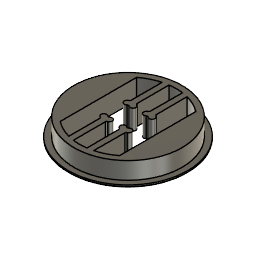
shifter bracket_v1 (Autodesk Fusion 360 design; units mm, degrees)
Autodesk Fusion 360 part; units mm, degrees
note: some values were not read from the file. Set by a fixed rule: which sketch regions a step uses.
sketch "Sketch1" plane through (0, 0, 0) normal (0, 0, 1) x (1, 0, 0)
  circle A0 centre (0, 0) radius 21
  dimension "d1" = 42
  constraint coincident A0.centre origin
  measures "d1" diameter of A0
extrude "Extrude1" add sketch "Sketch1" along normal blind 1
sketch "Sketch2" plane through (0, 0, 1) normal (0, 0, 1) x (-1, 0, 0)
  circle A0 centre (0, 0) radius 21
  circle A1 centre (0, 0) radius 19
  dimension "d4" = 38
  constraint coincident A0.centre A1.centre
  measures "d4" diameter of A1
extrude "Extrude2" add sketch "Sketch2" along normal blind 6 contours A1
sketch "Sketch3" plane through (0, 0, 7) normal (0, 0, 1) x (-1, 0, 0)
  circle A0 centre (0, 0) radius 19
  circle A1 centre (0, 0) radius 2 construction
  line L0 (4.4074, 16.8232) -> (4.4074, 5.4989)
  line L1 (2.372, 5.5528) -> (2.372, 17.2616)
  line L2 (0, 0) -> (0, 17.8293) construction
  line L3 (-4.3475, 16.841) -> (-4.4034, 5.4975)
  line L4 (-2.3033, 5.524) -> (-2.372, 17.2616)
  arc A2 (-3.0182, 3.3969) -> (-1.9879, 5.0695) centre (-2.3432, 4.1347) ccw
  arc A3 (-4.736, 5.035) -> (-3.7057, 3.3816) centre (-4.413, 4.0885) ccw
  arc A4 (3.7057, 3.3816) -> (4.7389, 5.034) centre (4.413, 4.0885) ccw
  arc A5 (2.0329, 5.0854) -> (3.0182, 3.3969) centre (2.3432, 4.1347) ccw
  line L5 (8.974, 0) -> (-11.026, 0) construction
  line L6 (-10.4146, 13.4129) -> (-10.4146, -13.4129)
  circle A6 centre (0, 0) radius 2 construction
  line L7 (10.4146, 13.4129) -> (10.4146, -13.4129)
  arc A7 (-3.0182, 3.3969) -> (-3.7057, 3.3816) centre (-3.354, 3.03) ccw
  arc A8 (-2.3033, 5.524) -> (-1.9879, 5.0695) centre (-1.8141, 5.5268) ccw
  arc A9 (-4.736, 5.035) -> (-4.4034, 5.4975) centre (-4.8947, 5.4999) ccw
  arc A10 (2.0329, 5.0854) -> (2.372, 5.5528) centre (1.8803, 5.5528) ccw
  arc A11 (3.7057, 3.3816) -> (3.0182, 3.3969) centre (3.354, 3.03) ccw
  arc A12 (4.4074, 5.4989) -> (4.7389, 5.034) centre (4.8991, 5.4989) ccw
  arc A13 (-4.4034, -5.4975) -> (-4.736, -5.035) centre (-4.8947, -5.4999) ccw
  arc A14 (-1.9879, -5.0695) -> (-3.0182, -3.3969) centre (-2.3432, -4.1347) ccw
  arc A15 (-1.9879, -5.0695) -> (-2.3033, -5.524) centre (-1.8141, -5.5268) ccw
  arc A16 (3.0182, -3.3969) -> (2.0329, -5.0854) centre (2.3432, -4.1347) ccw
  arc A17 (3.0182, -3.3969) -> (3.7057, -3.3816) centre (3.354, -3.03) ccw
  arc A18 (4.7389, -5.034) -> (3.7057, -3.3816) centre (4.413, -4.0885) ccw
  arc A19 (-3.7057, -3.3816) -> (-4.736, -5.035) centre (-4.413, -4.0885) ccw
  arc A20 (2.372, -5.5528) -> (2.0329, -5.0854) centre (1.8803, -5.5528) ccw
  arc A21 (-3.7057, -3.3816) -> (-3.0182, -3.3969) centre (-3.354, -3.03) ccw
  arc A22 (4.7389, -5.034) -> (4.4074, -5.4989) centre (4.8991, -5.4989) ccw
  line L8 (4.4074, -16.8232) -> (4.4074, -5.4989)
  line L9 (2.372, -5.5528) -> (2.372, -17.2616)
  line L10 (-2.3033, -5.524) -> (-2.372, -17.2616)
  line L11 (-4.3475, -16.841) -> (-4.4034, -5.4975)
  circle A23 centre (0, 0) radius 16.9815
  point P0 (0, 10.0735)
  point P1 (0, -10.0735)
  dimension "d7" = 4
  dimension "d9" = 2
  dimension "d14" = 2
  constraint coincident A0.centre A1.centre
  constraint vertical L0
  constraint vertical L1
  constraint vertical L2
  constraint coincident L2 P0
  constraint symmetric L1.end L2 L4.end
  constraint symmetric L2 A2 A5
  constraint symmetric L2 A3 A4
  constraint horizontal L5
  constraint vertical L6
  constraint symmetric A1 L2 A6
  constraint symmetric L2 L6.start L7.start
  constraint symmetric L2 L6.end L7.end
  constraint tangent A2 A7
  constraint tangent A3 A7
  constraint tangent A2 A8
  constraint tangent L4 A8
  constraint tangent L3 A9
  constraint tangent A3 A9
  constraint tangent A5 A10
  constraint tangent L1 A10
  constraint tangent A4 A11
  constraint tangent A5 A11
  constraint tangent A4 A12
  constraint tangent L0 A12
  constraint symmetric P0 L5 P1
  constraint symmetric A2 L5 A14
  constraint symmetric A3 L5 A19
  constraint symmetric A4 L5 A18
  constraint symmetric A5 L5 A16
  constraint symmetric L5 A2.start A14.end
  constraint symmetric L5 A3.end A19.start
  constraint symmetric L5 A7 A21
  constraint symmetric L5 L4.start A15.end
  constraint symmetric L5 A2.end A14.start
  constraint symmetric L5 A8 A15
  constraint symmetric L5 L3.end A13.start
  constraint symmetric L5 A3.start A13.end
  constraint symmetric L5 A9 A13
  constraint symmetric L5 L1.start A20.start
  constraint symmetric L5 A5.start A16.end
  constraint symmetric L5 A10 A20
  constraint symmetric L5 A4.start A17.end
  constraint symmetric L5 A5.end A16.start
  constraint symmetric L5 A11 A17
  constraint symmetric L5 L0.end A22.end
  constraint symmetric L5 A4.end A18.start
  constraint symmetric L5 A12 A22
  constraint symmetric L1.end L5 L9.end
  constraint symmetric L4.end L5 L10.end
  constraint symmetric L5 L0.start L8.start
  constraint symmetric L5 L3.start L11.start
  constraint coincident L5 A0.centre
  constraint coincident L6.end A23
  measures "d7" diameter of A1
  measures "d9" diameter of A5
  measures "d14" diameter of A4
extrude "Extrude3" cut sketch "Sketch3" against normal blind 11 contours L0 L1 L3 L4 A2 A3 A4 A5 L6 L7 A7 A8 A9 A10 A11 A12 A13 A14 A15 A16 A17 A18 A19 A20 A21 A22 L8 L9 L10 L11 A23
chamfer "Chamfer1" distance 0.5 angle 45 1 edges at (-19.5789, -7.5939, 0)
